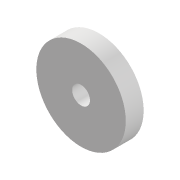
# Autodesk Inventor part: 大齿轮
Saved by Autodesk Inventor 2022 (Build 260153000, 153)
## iProperties
Created: 2023-03-19
Part Number: 大齿轮
Material: 常规
Document SubType Name: Modeling
Designer: Lzy18
Density: 1 g/cm^3
Appearance: 默认
Author: Lzy18
Autodesk Inventor part; units mm, degrees
ref_plane "YZ Plane" through (0, 0, 0) normal (1, 0, 0) x (0, 1, 0)
ref_plane "XZ Plane" through (0, 0, 0) normal (0, 1, 0) x (-1, 0, 0)
ref_plane "XY Plane" through (0, 0, 0) normal (0, 0, 1) x (1, 0, 0)
sketch "草图1" plane through (0, 0, 0) normal (0, 0, 1) x (1, 0, 0)
  circle A0 centre (-11.6139, -15) radius 1.5 projected
  circle A1 centre (-11.6139, 30) radius 1.5 projected
  circle A2 centre (-11.6139, -30) radius 1.5 projected
  circle A3 centre (-11.6139, 0) radius 1.5 projected
  circle A4 centre (-11.6139, 15) radius 1.5 projected
  circle A5 centre (4.1139, -46.09) radius 2.5 projected
  circle A6 centre (4.1139, 46.09) radius 2.5 projected
  arc A7 (14.6139, -69.4727) -> (19.1139, -66.8746) centre (16.1139, -66.8746) ccw projected
  line L0 (19.1139, -66.8746) -> (19.1139, -60.9783) projected
  line L1 (19.1139, -60.9783) -> (7.115, -57.7054) projected
  line L2 (7.115, -57.7054) -> (7.115, 54.3279) projected
  line L3 (7.115, 54.3279) -> (19.1139, 59.6306) projected
  line L4 (19.1139, 59.6306) -> (19.1139, 66.8746) projected
  arc A8 (19.1139, 66.8746) -> (14.6139, 69.4727) centre (16.1139, 66.8746) ccw projected
  line L5 (14.6139, 69.4727) -> (-17.6139, 50.866) projected
  arc A9 (-17.6139, 50.866) -> (-19.1139, 48.2679) centre (-16.1139, 48.2679) ccw projected
  line L6 (-19.1139, 48.2679) -> (-19.1139, -48.2679) projected
  arc A10 (-19.1139, -48.2679) -> (-17.6139, -50.866) centre (-16.1139, -48.2679) ccw projected
  line L7 (-17.6139, -50.866) -> (14.6139, -69.4727) projected
  circle A11 centre (4.1139, 46.09) radius 12.5
  point P0 (0, 0)
  dimension "d0" = 25
  constraints: 1 centre point, 1 coincident
  measures "d0" diameter of A11
extrude "拉伸1" add sketch "草图1" along normal blind 5 contours A11 L3 L2 | L2 L3 A11
